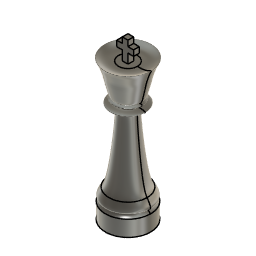
king (Autodesk Fusion 360 design; units mm, degrees)
Autodesk Fusion 360 part; units mm, degrees
sketch "Profile" plane through (0, 0, 0) normal (0, 1, 0) x (1, 0, 0)
  line L0 (4.127, 0) -> (12.7, 0)
  line L1 (0, -8.1) -> (0, -88.9)
  line L2 (4.127, -8.1) -> (4.127, 0)
  line L3 (4.127, -8.1) -> (0, -8.1)
  line L4 (12.7, 0) -> (12.7, -8.89)
  spline S0 degree 5 poles (5.3405, -55.017) (5.3762, -55.0492) (5.4478, -55.115) (5.5558, -55.2182) (5.7133, -55.3591) (5.9669, -55.5137) (6.2991, -55.6233) (6.621, -55.6859) (6.8259, -55.7322) (7.0347, -55.7959) (7.3932, -55.9108) (8.0147, -56.098) (8.8644, -56.3583) (9.6586, -56.6604) (10.0183, -56.9566) (9.7065, -57.2022) (8.7248, -57.3688) (7.7497, -57.4735) (7.0872, -57.5362) (6.7459, -57.5747) (6.5617, -57.6055) (6.3427, -57.6344) (6.0362, -57.6625) (5.7541, -57.6845) (5.5936, -57.6963) knots 0 0 0 0 0 0 0.05 0.1 0.15 0.2 0.25 0.3 0.35 0.4 0.45 0.5 0.55 0.6 0.65 0.7 0.75 0.8 0.85 0.9 0.95 1 1 1 1 1 1
  line L5 (11.0344, -56.9344) -> (7.112, -57.658)
  line L6 (7.422, -57.5615) -> (3.7651, -57.8312)
  spline S1 degree 5 poles (10.7494, -15.8342) (10.6284, -15.9825) (10.3877, -16.3328) (10.0303, -17.0186) (9.561, -18.2564) (8.9874, -20.3467) (8.4293, -22.9668) (7.8907, -26.0702) (7.3783, -29.5575) (6.9004, -33.2926) (6.4666, -37.1181) (6.0867, -40.8697) (5.7704, -44.3899) (5.5255, -47.5422) (5.3576, -50.2263) (5.2682, -52.3947) (5.259, -53.706) (5.2864, -54.4529) (5.3199, -54.8464) (5.3405, -55.017) knots 0 0 0 0 0 0 0.066667 0.133333 0.2 0.266667 0.333333 0.4 0.466667 0.533333 0.6 0.666667 0.733333 0.8 0.866667 0.933333 1 1 1 1 1 1
  spline S2 degree 5 poles (12.7, -8.89) (12.5424, -9.007) (12.2481, -9.2311) (11.8699, -9.538) (11.4927, -9.8882) (11.2346, -10.2278) (11.1833, -10.4749) (11.3186, -10.6439) (11.5969, -10.7641) (11.9494, -10.8801) (12.2992, -11.041) (12.5722, -11.2938) (12.7141, -11.6719) (12.6933, -12.1936) (12.4938, -12.867) (12.1099, -13.6936) (11.6558, -14.4758) (11.234, -15.1293) (10.9169, -15.5943) (10.7494, -15.8342) knots 0 0 0 0 0 0 0.066667 0.133333 0.2 0.266667 0.333333 0.4 0.466667 0.533333 0.6 0.666667 0.733333 0.8 0.866667 0.933333 1 1 1 1 1 1
  line L7 (4.5578, -54.3126) -> (6.1231, -55.7214)
  spline S3 degree 5 poles (5.5936, -57.6963) (5.5048, -57.7363) (5.3437, -57.8116) (5.1517, -57.9102) (4.9948, -58.0131) (4.9621, -58.0982) (5.0873, -58.1517) (5.3587, -58.1978) (5.756, -58.2655) (6.2475, -58.3795) (6.7875, -58.552) (7.3121, -58.7726) (7.7504, -59.0151) (8.0384, -59.2478) (8.1323, -59.4424) (8.0216, -59.5835) (7.7433, -59.6784) (7.3663, -59.7471) (6.975, -59.8134) (6.6533, -59.8926) (6.4683, -59.9878) (6.4579, -60.097) (6.6119, -60.2171) (6.8716, -60.349) (7.1634, -60.4989) (7.429, -60.6816) (7.6491, -60.9211) (7.8283, -61.2439) (7.9858, -61.6734) (8.1439, -62.2237) (8.3165, -62.8931) (8.5088, -63.666) (8.7192, -64.5168) (8.9417, -65.4135) (9.1672, -66.3214) (9.3855, -67.2063) (9.5871, -68.0388) (9.765, -68.7972) (9.9164, -69.4711) (10.0451, -70.0662) (10.1599, -70.6007) (10.2722, -71.1002) (10.394, -71.5923) (10.5355, -72.1016) (10.7028, -72.6446) (10.8954, -73.2244) (11.1056, -73.8278) (11.3217, -74.433) (11.5308, -75.014) (11.7219, -75.547) (11.8886, -76.0155) (12.0321, -76.4156) (12.1646, -76.7632) (12.305, -77.0876) (12.4691, -77.4175) (12.6625, -77.7703) (12.8712, -78.1386) (13.0557, -78.4817) (13.1662, -78.7468) (13.1545, -78.8852) (12.9895, -78.8737) (12.6648, -78.7255) (12.192, -78.4763) (11.5957, -78.1751) (10.9078, -77.8725) (10.162, -77.6111) (9.3887, -77.4135) (8.6133, -77.2846) (7.8577, -77.2167) (7.1392, -77.1937) (6.4714, -77.1953) (5.9853, -77.2002) (5.6505, -77.1989) (5.4407, -77.195) (5.3391, -77.1922) knots 0 0 0 0 0 0 0.01428571 0.02857143 0.04285714 0.05714286 0.07142857 0.08571429 0.1 0.11428571 0.12857143 0.14285714 0.15714286 0.17142857 0.18571429 0.2 0.21428571 0.22857143 0.24285714 0.25714286 0.27142857 0.28571429 0.3 0.31428571 0.32857143 0.34285714 0.35714286 0.37142857 0.38571429 0.4 0.41428571 0.42857143 0.44285714 0.45714286 0.47142857 0.48571429 0.5 0.51428571 0.52857143 0.54285714 0.55714286 0.57142857 0.58571429 0.6 0.61428571 0.62857143 0.64285714 0.65714286 0.67142857 0.68571429 0.7 0.71428571 0.72857143 0.74285714 0.75714286 0.77142857 0.78571429 0.8 0.81428571 0.82857143 0.84285714 0.85714286 0.87142857 0.88571429 0.9 0.91428571 0.92857143 0.94285714 0.95714286 0.97142857 0.98571429 1 1 1 1 1 1
  line L8 (7.8063, -77.2589) -> (2.872, -77.1255)
  line L9 (5.3391, -77.1922) -> (0, -77.1922)
  line L10 (5.1776, -55.3266) -> (7.5224, -55.9254)
  point P0 (11.2931, -10.578)
  point P1 (12.4284, -11.1867)
  point P2 (9.0732, -57.2962)
  point P3 (8.128, -56.134)
  point P4 (6.8316, -57.15)
  point P5 (5.548, -47.3796)
  point P6 (8.4175, -23.1744)
  point P7 (5.0055, -58.0958)
  point P8 (6.4845, -60.0627)
  point P9 (10.6526, -72.475)
  point P10 (9.8012, -68.963)
  point P11 (13.1358, -78.8248)
  point P12 (6.35, -55.626)
  point P13 (6.35, -58.42)
  point P14 (8.0812, -59.4349)
  point P15 (7.1376, -59.7878)
  point P16 (7.1032, -60.4752)
  point P17 (8.0175, -61.8033)
  point P18 (10.7778, -77.8382)
  point P19 (11.9296, -76.1288)
  point P20 (12.6391, -77.7251)
  dimension "d1" = 12.7
  dimension "d2" = 88.9
  dimension "d5" = 8.89
  dimension "d9" = 4.127
  dimension "d10" = 8.1
  constraint horizontal L0
  constraint perpendicular L0 L1
  constraint perpendicular L0 L2
  constraint perpendicular L1 L3
  constraint perpendicular L0 L4
  constraint midpoint P2 L5
  constraint midpoint S0.end L6
  constraint coincident S1.start S2.end
  constraint midpoint S0.start L7
  constraint midpoint S3.end L8
  constraint coincident L1 L9.end
  constraint perpendicular L1 L9
  constraint midpoint P12 L10
  measures "d1" distance of origin L0.end
  measures "d2" distance of origin L1.end
  measures "d5" distance of L0.end L4.end
  measures "d9" distance of L1.start L2.start
  measures "d10" distance of L0.start L2.start
revolve "Revolve1" add sketch "Profile" angle 360 about axis through (0, 0, 8.1) along (0, 0, 1)
sketch "Cross" plane through (0, 0, 0) normal (0, 1, 0) x (1, 0, 0)
  line L0 (0, -88.9) -> (1.5875, -88.9)
  line L1 (1.5875, -88.9) -> (1.5875, -85.725)
  line L2 (1.5875, -85.725) -> (4.7625, -85.725)
  line L3 (4.7625, -85.725) -> (4.7625, -82.55)
  line L4 (4.7625, -82.55) -> (1.5875, -82.55)
  line L5 (5.3391, -77.1922) -> (0, -77.1922)
  line L6 (1.5875, -82.55) -> (1.5875, -77.1922)
  line L7 (0, -8.1) -> (0, -88.9)
  line L8 (-1.5875, -82.55) -> (-1.5875, -77.1922)
  line L9 (-4.7625, -82.55) -> (-1.5875, -82.55)
  line L10 (-4.7625, -85.725) -> (-4.7625, -82.55)
  line L11 (-1.5875, -85.725) -> (-4.7625, -85.725)
  line L12 (-1.5875, -88.9) -> (-1.5875, -85.725)
  line L13 (0, -88.9) -> (-1.5875, -88.9)
  line L14 (1.5875, -77.1922) -> (-1.5875, -77.1922)
  dimension "d38" = 1.5875
  dimension "d39" = 3.175
  dimension "d40" = 3.175
  dimension "d41" = 3.175
  dimension "d42" = 3.175
  constraint horizontal L0
  constraint perpendicular L0 L1
  constraint perpendicular L1 L2
  constraint perpendicular L2 L3
  constraint perpendicular L3 L4
  constraint coincident L5 L6.end
  constraint perpendicular L5 L6
  constraint symmetric L0.start L7 L13.start
  constraint symmetric L0.end L7 L12.start
  constraint symmetric L1.end L7 L11.start
  constraint symmetric L2.end L7 L10.start
  constraint symmetric L3.end L7 L9.start
  constraint symmetric L4.end L7 L8.start
  constraint symmetric L6.end L7 L8.end
  measures "d38" distance of L0.start L0.end
  measures "d39" distance of L0.end L1.end
  measures "d40" distance of L1.end L2.end
  measures "d41" distance of L2.end L3.end
  measures "d42" distance of L3.end L4.end
extrude "Extrude6" add sketch "Cross" along normal mid plane 3.175
